m3_nut (Autodesk Fusion 360 design; units mm, degrees)
Autodesk Fusion 360 part; units mm, degrees
sketch "Sketch1" plane through (0, 0, 0) normal (0, 1, 0) x (1, 0, 0)
  line L0 (-1.7321, -3) -> (1.7321, -3)
  line L1 (1.7321, -3) -> (3.4641, 0)
  line L2 (3.4641, 0) -> (1.7321, 3)
  line L3 (1.7321, 3) -> (-1.7321, 3)
  line L4 (-1.7321, 3) -> (-3.4641, 0)
  line L5 (-3.4641, 0) -> (-1.7321, -3)
  line L6 (-1.7321, -3) -> (1.7321, 3)
  line L7 (-1.7321, 3) -> (1.7321, -3)
  line L8 (3.4641, 0) -> (-3.4641, 0)
  dimension "d1" = 120
  dimension "d2" = 120
  dimension "d3" = 6
  dimension "d4" = 6
  dimension "d5" = 6
  constraint horizontal L0
  constraint parallel L0 L3
  constraint parallel L1 L4
  constraint parallel L2 L5
  constraint midpoint L6 L8
  constraint midpoint origin L6
  measures "d1" angle of L1 L2
  measures "d2" angle of L0 L1
  measures "d3" distance of L0 L3
  measures "d4" distance of L1 L4
  measures "d5" distance of L2 L5
extrude "Extrude1" add sketch "Sketch1" along normal blind 2.25
equation "d3 = d4"
equation "d5 = d4"
